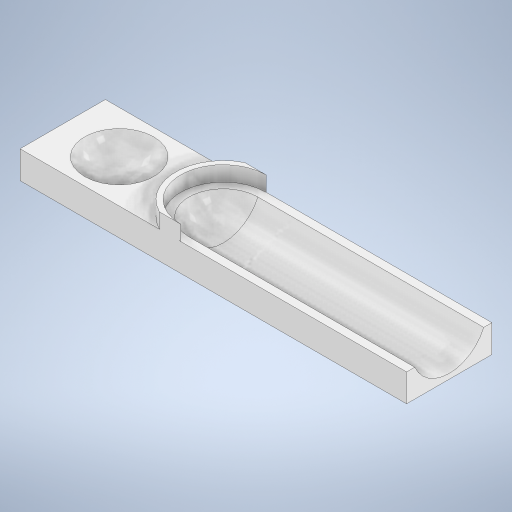
# Autodesk Inventor part: Trilho 60 minutos  - 12 horas
Saved by Autodesk Inventor 2024 (Build 280153000, 153)
## iProperties
Created: 2023-05-09
Part Number: Trilho 60 minutos  - 12 horas
Material: Plástico PET
Document SubType Name: Modeling
Designer: jpjoa
Density: 1.541 g/cm^3
Appearance: Branco
Author: jpjoa
Autodesk Inventor part; units mm, degrees
ref_plane "YZ Plane" through (0, 0, 0) normal (1, 0, 0) x (0, 1, 0)
ref_plane "XZ Plane" through (0, 0, 0) normal (0, 1, 0) x (-1, 0, 0)
ref_plane "XY Plane" through (0, 0, 0) normal (0, 0, 1) x (1, 0, 0)
sketch "Esboço2" plane through (0, 0, 0) normal (0, 1, 0) x (-1, 0, 0)
  line L0 (-33.3088, 0) -> (-92.4, 0)
  line L1 (-92.4, 0) -> (-92.4, -20.4)
  line L2 (-92.4, -20.4) -> (-33.3088, -20.4)
  line L3 (-38.4, -19.2) -> (-92.4, -19.2)
  line L4 (-92.4, -1.2) -> (-38.4, -1.2)
  circle A0 centre (-38.4, -10.2) radius 9
  line L5 (-47.4, -20.4) -> (-47.4, -19.2)
  line L6 (-47.4, -1.2) -> (-47.4, 0)
  arc A1 (-33.3088, -20.4) -> (-33.3088, 0) centre (-38.4, -10.2) ccw
  arc A2 (-38.4, -20.4) -> (-38.4, 0) centre (-38.4, -10.2) ccw
  line L7 (-33.3088, 0) -> (0, 0)
  line L8 (0, 0) -> (0, -20.4)
  line L9 (0, -20.4) -> (-33.3088, -20.4)
  circle A3 centre (-13.5, -10.2) radius 9
  point P0 (0, -10.2)
  point P1 (-33.3088, -20.4)
  dimension "d6" = 20.4
  dimension "d8" = 1.2
  dimension "d11" = 1.2
  dimension "d25" = 18
  dimension "d44" = 1.2
  dimension "d45" = 1.2
  dimension "d46" = 54
  dimension "d47" = 27
  dimension "d48" = 18
  dimension "d49" = 13.5
  constraints: 20 end point, 8 point on line, 6 point on circle, 5 perpendicular, 4 centre point, 3 tangent, 2 horizontal, 2 horizontal alignment, 2 vertical, 1 coincident, 1 midpoint
  measures "d6" distance of L0.end L1.end
  measures "d8" distance between parallel lines of L2 L3
  measures "d11" distance between parallel lines of L0 L4
  measures "d25" diameter of A0
  measures "d44" radial gap between concentric circles of A2 A1
  measures "d45" radial gap between concentric circles of A0 A2
  measures "d46" distance from line of L1 A0.centre
  measures "d47" distance edge to line of A1 L8
  measures "d48" diameter of A3
  measures "d49" distance from line of L8 A3.centre
extrude "Extrusão1" add sketch "Esboço2" against normal blind 1.2 contours A1 L2 A2 L0 | L7 L8 L9 A1 | A2 L2 L5 L3 A0 L4 L6 L0 | L6 L4 L1 L0 | L4 A0 L3 L1 | L2 L1 L3 L5 | A0 | A3
extrude "Extrusão2" add sketch "Esboço2" along normal blind 9 contours L7 L8 L9 A1 | A2 L2 L5 L3 A0 L4 L6 L0 | L6 L4 L1 L0 | L2 L1 L3 L5
fillet "Arredondamento6" radius 9 4 edges at (65.4, 0, -1.2) (65.4, 0, -19.2) (29.4, 0, -10.2) (22.5, 0, -10.2)
sketch "Esboço6" plane through (0, -1.2, 0) normal (0, 0, 1) x (1, 0, 0)
  line L0 (92.4, 10.2) -> (0, 10.2)
  line L1 (0, 10.2) -> (0, 6.6)
  line L2 (0, 6.6) -> (92.4, 6.6)
  line L3 (92.4, 6.6) -> (92.4, 10.2)
  line L4 (92.4, 1.2) -> (92.4, 10.2) projected
  line L5 (0, 10.2) -> (0, 0) projected
  line L6 (38.4, 10.2) -> (92.4, 10.2) projected
  line L7 (38.4, 1.2) -> (92.4, 1.2) projected
  point P0 (0, 1.2)
  point P1 (92.4, 8.4)
  point P2 (92.4, 5.7)
  point P3 (0, 8.4)
  point P4 (0, 5.1)
  point P5 (46.2, 10.2)
  point P6 (65.4, 10.2)
  dimension "d50" = 5.4
  constraints: 8 end point, 6 midpoint, 2 perpendicular, 2 vertical alignment, 1 horizontal, 1 horizontal alignment, 1 vertical
  measures "d50" distance between parallel lines of L7 L2
extrude "Extrusão8" cut sketch "Esboço6" against normal up to surface (20.4 mm away)
extrude "Extrusão9" add sketch "Esboço2" along normal blind 9 contours A1 L2 A2 L0
sketch "Esboço7" plane through (0, -1.2, 0) normal (0, -1, 0) x (1, 0, 0)
  line L0 (42.3, -11.4) -> (50.1, -11.4)
  line L1 (50.1, -11.4) -> (50.1, -9)
  line L2 (50.1, -9) -> (42.3, -9)
  line L3 (42.3, -9) -> (42.3, -11.4)
  line L4 (0, 0) -> (0, -20.4) projected
  arc A0 (38.4, 0) -> (38.4, -20.4) centre (38.4, -10.2) ccw projected
  line L5 (92.4, -20.4) -> (92.4, 0) projected
  point P0 (42.3, -10.2)
  point P1 (0, -10.2)
  point P2 (46.2, -9)
  point P3 (28.2, -10.2)
  dimension "d56" = 7.8
  dimension "d57" = 2.4
  dimension "d76" = 42.3
  dimension "d77" = 42.3
  constraints: 8 end point, 3 midpoint, 3 perpendicular, 1 horizontal, 1 horizontal alignment, 1 point on circle
  measures "d56" distance of L0.start L0.end
  measures "d57" distance of L0.end L1.end
  measures "d76" distance between parallel lines of L4 L3
  measures "d77" distance between parallel lines of L5 L1
extrude "Extrusão10" add sketch "Esboço7" along normal blind 5.4
sketch "Esboço8" plane through (42.3, -1.2, -9) normal (0, 0, 1) x (1, 0, 0)
  circle A0 centre (3.9, -2.7) radius 1.5
  line L0 (50.1, 0) -> (-42.3, 0) projected
  line L1 (7.8, 0) -> (7.8, -5.4)
  line L2 (0, 0) -> (0, -5.4)
  line L3 (7.8, -5.4) -> (0, -5.4) projected
  line L4 (7.8, -5.4) -> (0, -5.4)
  arc A1 (1.2, -2.7) -> (6.6, -2.7) centre (3.9, -2.7) ccw
  line L5 (1.2, -2.7) -> (1.2, -1.2)
  line L6 (6.6, -2.7) -> (6.6, -1.2)
  line L7 (0, 0) -> (0, 0)
  line L8 (7.8, 0) -> (7.8, 0)
  arc A2 (1.2, -1.2) -> (0, 0) centre (0, -1.2) ccw
  arc A3 (7.8, 0) -> (6.6, -1.2) centre (7.8, -1.2) ccw
  line L9 (0, 0) -> (7.8, 0) projected
  point P0 (-42.3, 1.2)
  point P1 (3.9, 0)
  point P2 (1.2, 0)
  point P3 (6.6, 0)
  point P4 (1.2, 0)
  point P5 (6.6, 0)
  point P6 (3.9, -5.4)
  point P7 (3.9, 0)
  dimension "d60" = 3
  dimension "d61" = 2.7
  dimension "d63" = 1.2
  dimension "d64" = 1.2
  constraints: 14 end point, 14 midpoint, 8 coincident, 6 horizontal alignment, 6 point on circle, 6 tangent, 4 centre point, 4 point on line, 3 horizontal, 3 vertical, 1 equal radius, 1 perpendicular, 1 vertical alignment
  measures "d60" diameter of A0
  measures "d61" distance from line of L0 A0.centre
  measures "d63" radial gap between concentric circles of A1 A0
  measures "d64" radius of A2
extrude "Extrusão11" cut sketch "Esboço8" against normal up to surface (2.4 mm away) contours A0 | L1 L3 A1 L6 A3 | A2 L5 A1 L3 L2
equation "\"d6\" = Diâmetro_esfera + 2 * Margem"
equation "\"d8\" = Margem"
equation "\"d11\" = Margem"
equation "\"d25\" = Diâmetro_esfera"
equation "\"d44\" = Margem"
equation "\"d45\" = Margem"
equation "\"d46\" = 3 * Diâmetro_esfera"
equation "\"d48\" = Diâmetro_esfera"
equation "\"d49\" = 0.5 * d47"
equation "\"d13\" = Margem"
equation "\"d15\" = 0.5 * Diâmetro_esfera"
equation "\"d55\" = 0.5 * Diâmetro_esfera"
equation "\"d50\" = 0.3 * Diâmetro_esfera"
equation "\"d53\" = 0.5 * Diâmetro_esfera"
equation "\"d56\" = Parafuso + 4 * Margem"
equation "\"d57\" = 2 * Margem"
equation "\"d58\" = Parafuso + 2 * Margem"
equation "\"d60\" = Parafuso"
equation "\"d61\" = 0.5 * Parafuso + Margem"
equation "\"d63\" = Margem"
equation "\"Diâmetro_esfera\" = 18"
equation "\"Margem\" = 3 * Filamento"
equation "\"Filamento\" = 0.4"
equation "\"Parafuso\" = 3"
equation "\"d42\" = Margem"
equation "\"d43\" = Margem"
equation "\"Tamanho_receptor\" = 37.257"
